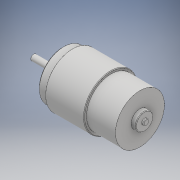
# Autodesk Inventor part: RS-775
Saved by Autodesk Inventor 2017 (Build 210142000, 142)
## iProperties
Part Number: RS-775
Material: 一般
Document SubType Name: Modeling
Designer: highs
Density: 1 g/cm^3
Appearance: 既定
Author: highs
Autodesk Inventor part; units mm, degrees
ref_plane "YZ Plane" through (0, 0, 0) normal (1, 0, 0) x (0, 1, 0)
ref_plane "XZ Plane" through (0, 0, 0) normal (0, 1, 0) x (-1, 0, 0)
ref_plane "XY Plane" through (0, 0, 0) normal (0, 0, 1) x (1, 0, 0)
sketch "スケッチ1" plane through (0, 0, 0) normal (0, 0, 1) x (1, 0, 0)
  line L0 (20.8, 7.5) -> (25, 7.5)
  line L1 (25, 7.5) -> (25, 21.05)
  line L2 (25, 21.05) -> (33, 21.05)
  line L3 (33, 21.05) -> (33, 23.15)
  line L4 (33, 23.15) -> (66.6, 23.15)
  line L5 (66.6, 23.15) -> (66.6, 21.05)
  line L6 (66.6, 21.05) -> (91.5, 21.05)
  line L7 (91.5, 21.05) -> (91.5, 7.5)
  line L8 (91.5, 7.5) -> (95.5, 7.5)
  line L9 (95.5, 7.5) -> (95.5, 2.5)
  line L10 (95.5, 2.5) -> (97, 2.5)
  line L11 (97, 2.5) -> (97, 0)
  line L12 (97, 0) -> (0, 0)
  line L13 (20.8, 7.5) -> (20.8, 2.5)
  line L14 (20.8, 2.5) -> (0, 2.5)
  line L15 (0, 2.5) -> (0, 0)
  dimension "d1" = 4.2
  dimension "d2" = 21.05
  dimension "d3" = 23.15
  dimension "d4" = 8
  dimension "d5" = 33.6
  dimension "d6" = 66.5
  dimension "d7" = 7.5
  dimension "d8" = 4
  dimension "d9" = 7.5
  dimension "d10" = 97
  dimension "d11" = 25
  dimension "d12" = 2.5
  dimension "d13" = 2.5
  constraints: 32 end point, 12 perpendicular, 2 point on line, 1 vertical
  measures "d1" distance of L0.start L0.end
  measures "d2" distance between parallel lines of L12 L2
  measures "d3" distance between parallel lines of L12 L4
  measures "d4" distance of L1.end L2.end
  measures "d5" distance of L3.end L4.end
  measures "d6" distance between parallel lines of L7 L1
  measures "d7" distance between parallel lines of L12 L8
  measures "d8" distance of L7.end L8.end
  measures "d9" distance between parallel lines of L12 L0
  measures "d10" distance between parallel lines of L11 L15
  measures "d11" distance between parallel lines of L1 L15
  measures "d12" distance between parallel lines of L12 L14
  measures "d13" distance between parallel lines of L12 L10
revolve "回転1" add sketch "スケッチ1" angle 360 about axis through (97, 0, 0) along (-1, 0, 0)
chamfer "面取り1" distance 1 angle 45 1 edges at (25, -21.05, 0)
fillet "フィレット1" radius 0.5 4 edges at (33, -23.15, 0) (66.6, -23.15, 0) (95.5, -7.5, 0) (97, -2.5, 0)
